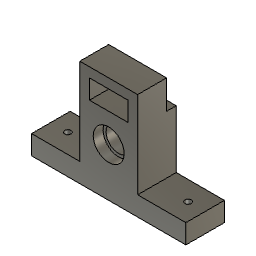
Base structure with cable holder (Autodesk Fusion 360 design; units mm, degrees)
Autodesk Fusion 360 part; units mm, degrees
sketch "Esquisse1" plane through (0, 0, 0) normal (0, 0, 1) x (1, 0, 0)
  line L0 (-40, 10) -> (40, 10)
  line L1 (40, 10) -> (40, -10)
  line L2 (40, -10) -> (-40, -10)
  line L3 (-40, -10) -> (-40, 10)
  constraint horizontal L0
  constraint vertical L1
  constraint horizontal L2
  constraint vertical L3
extrude "Extrusion1" add sketch "Esquisse1" along normal blind 10
sketch "Esquisse2" plane through (0, 0, 10) normal (0, 0, 1) x (-1, 0, 0)
  line L0 (40, 10) -> (-40, 10)
  line L1 (-40, 10) -> (-40, -10)
  line L2 (-40, -10) -> (40, -10)
  line L3 (40, -10) -> (40, 10)
  line L4 (15, -10) -> (-15, -10)
  line L5 (-15, -10) -> (-15, 10)
  line L6 (-15, 10) -> (15, 10)
  line L7 (15, 10) -> (15, -10)
  circle A0 centre (-31.183, 0) radius 1.625
  circle A1 centre (31.183, 0) radius 1.625
  dimension "d7" = 3.25
  dimension "d8" = 3.25
  constraint horizontal L4
  constraint vertical L5
  constraint horizontal L6
  constraint vertical L7
  constraint coincident L0 L5.end
  measures "d7" diameter of A0
  measures "d8" diameter of A1
extrude "Extrusion2" cut sketch "Esquisse2" against normal blind 10 contours A1
extrude "Extrusion3" cut sketch "Esquisse2" against normal blind 10 contours A0
extrude "Extrusion4" add sketch "Esquisse2" along normal blind 30 contours L0 L2 L4 L5 L6 L7
sketch "Esquisse3" plane through (0, -10, 0) normal (0, -1, 0) x (1, 0, 0)
  line L0 (-40, 0) -> (40, 0)
  line L1 (40, 0) -> (40, 10)
  line L2 (40, 10) -> (15, 10)
  line L3 (15, 10) -> (15, 40)
  line L4 (15, 40) -> (-15, 40)
  line L5 (-15, 40) -> (-15, 10)
  line L6 (-15, 10) -> (-40, 10)
  line L7 (-40, 10) -> (-40, 0)
  circle A0 centre (0, 25) radius 6.5
  circle A1 centre (0, 25) radius 8
  dimension "d15" = 13
  dimension "d16" = 16
  constraint concentric A0 A1
  measures "d15" diameter of A0
  measures "d16" diameter of A1
extrude "Extrusion5" cut sketch "Esquisse3" against normal blind 20 contours A0
extrude "Extrusion6" cut sketch "Esquisse3" against normal blind 5.1 contours A1
sketch "Esquisse4" plane through (0, 0, 40) normal (0, 0, 1) x (-1, 0, 0)
  line L0 (15, 10) -> (-15, 10)
  line L1 (-15, 10) -> (-15, -10)
  line L2 (-15, -10) -> (15, -10)
  line L3 (15, -10) -> (15, 10)
  line L4 (15, 10) -> (10, 10)
  line L5 (10, 10) -> (10, -5)
  line L6 (10, -5) -> (15, -5)
  line L7 (15, -5) -> (15, 10)
  line L8 (-15, 10) -> (-10, 10)
  line L9 (-10, 10) -> (-10, -5)
  line L10 (-10, -5) -> (-15, -5)
  line L11 (-15, -5) -> (-15, 10)
  constraint horizontal L4
  constraint vertical L5
  constraint horizontal L6
  constraint vertical L7
  constraint coincident L0.start L3.end
  constraint horizontal L8
  constraint vertical L9
  constraint horizontal L10
  constraint vertical L11
  constraint coincident L0.end L1.start
extrude "Extrusion7" add sketch "Esquisse4" along normal blind 10 contours L0 L3 L4 L5 L6 L7 | L0 L1 L8 L9 L10 L11
sketch "Esquisse5" plane through (0, 0, 50) normal (0, 0, 1) x (-1, 0, 0)
  line L0 (15, -5) -> (15, 10)
  line L1 (15, 10) -> (10, 10)
  line L2 (10, 10) -> (10, -5)
  line L3 (10, -5) -> (15, -5)
  line L4 (15, -5) -> (-15, -5)
  line L5 (-15, -5) -> (-15, 10)
  line L6 (-15, 10) -> (15, 10)
  line L7 (15, 10) -> (15, -5)
  constraint horizontal L4
  constraint vertical L5
  constraint horizontal L6
  constraint vertical L7
  constraint coincident L0.start L3.end
extrude "Extrusion8" add sketch "Esquisse5" along normal blind 5
